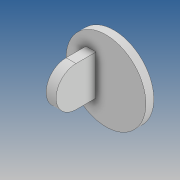
# Autodesk Inventor part: podstawa
Saved by Autodesk Inventor 2022.3 (Build 263350000, 350)
## iProperties
Created: 2023-06-25
Part Number: podstawa
Material: Ogólny
Document SubType Name: Modeling
Designer: Chyba Ja
Density: 1 g/cm^3
Appearance: Domyślna
Author: Chyba Ja
Autodesk Inventor part; units mm, degrees
ref_plane "YZ Plane" through (0, 0, 0) normal (1, 0, 0) x (0, 1, 0)
ref_plane "XZ Plane" through (0, 0, 0) normal (0, 1, 0) x (-1, 0, 0)
ref_plane "XY Plane" through (0, 0, 0) normal (0, 0, 1) x (1, 0, 0)
sketch "Szkic1" plane through (0, 0, 0) normal (0, 0, 1) x (1, 0, 0)
  circle A0 centre (0, 0) radius 50
  line L0 (-25, 25) -> (-12.5, 25)
  line L1 (-12.5, -25) -> (-25, -25)
  line L2 (-25, -25) -> (-25, 25)
  line L3 (-12.5, -25) -> (-12.5, 25)
  point P0 (-12.5, 0)
  point P1 (-18.75, 25)
  dimension "d0" = 100
  dimension "d10" = 12.5
  dimension "d11" = 12.5
  dimension "d12" = 50
  dimension "d13" = 25
  constraints: 8 end point, 2 midpoint, 1 centre point, 1 coincident, 1 horizontal, 1 parallel, 1 vertical
  measures "d0" diameter of A0
  measures "d10" distance of point (-12.5, 0) point (0, 0)
  measures "d11" distance between parallel lines of L2 L3
  measures "d12" distance from line of L1 point (-18.75, 25)
  measures "d13" distance centre to line of A0 L0
extrude "Wyciągnięcie proste1" add sketch "Szkic1" along normal blind 60 contours L0 L3 L1 L2
extrude "Wyciągnięcie proste2" add sketch "Szkic1" along normal blind 10 contours A0 | L0 L3 L1 L2
sketch "Szkic2" plane through (-25, -25, 60) normal (-1, 0, 0) x (0, 0, 1)
  line L0 (-50, 50) -> (-50, 0) projected
  line L1 (-50, 0) -> (0, 0) projected
  line L2 (0, 50) -> (0, 0) projected
  line L3 (-50, 50) -> (0, 50) projected
  circle A0 centre (-25, 25) radius 25
  line L4 (-50, 50) -> (0, 50) projected
  line L5 (0, 50) -> (0, 0) projected
  line L6 (-25, 50) -> (0, 50)
  line L7 (0, 25) -> (0, 0)
  point P0 (-60, 25)
  point P1 (-25, 50)
  point P2 (0, 25)
  point P3 (-25, 0)
  dimension "d7" = 50
  constraints: 4 end point, 4 tangent, 2 collinear, 2 midpoint, 1 centre point
  measures "d7" diameter of A0
extrude "Wyciągnięcie proste3" cut sketch "Szkic2" against normal through all contours L3 L2 A0 | A0 L2 L1
